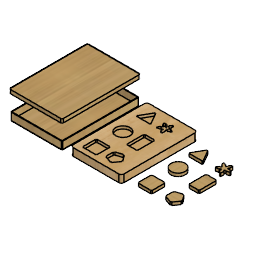
Modelação fushion_Parametrico (Autodesk Fusion 360 design; units mm, degrees)
Autodesk Fusion 360 part; units mm, degrees
sketch "Sketch1" plane through (0, 0, 0) normal (0, 1, 0) x (1, 0, 0)
sketch "Sketch2" plane through (0, 0, 0) normal (0, 0, 1) x (1, 0, 0)
  line L0 (0, 0) -> (-201, 0)
  line L1 (-201, 0) -> (-201, -301)
  line L2 (-201, -301) -> (0, -301)
  line L3 (0, -301) -> (0, 0)
  line L4 (1, -302) -> (1, 1)
  line L5 (1, 1) -> (-202, 1)
  line L6 (-202, 1) -> (-202, -302)
  line L7 (-202, -302) -> (1, -302)
  dimension "d11" = 201
  dimension "d12" = 301
  dimension "d13" = 1
  constraint horizontal L0
  constraint vertical L1
  constraint horizontal L2
  constraint vertical L3
  constraint coincident L0.start L3.end
  measures "d11" distance of L0.start L0.end
  measures "d12" distance of L0.start L2.end
extrude "Extrude1" add sketch "Sketch2" along normal blind 30 contours L0 L1 L2 L3 | L4 L5 L6 L7 makes body 1
fillet "Fillet1" radius 2.5 4 edges at (1, 1, 15) (1, -302, 15) (-202, 1, 15) (-202, -302, 15) on bodies 1
shell "Shell1" thickness 2.5 removed faces 1 at (-134.3333, -100.8333, 30) on bodies 1
sketch "Sketch3" plane through (0, 0, 30) normal (0, 0, 1) x (-1, 0, 0)
  line L0 (199.5, 1.5) -> (1.5, 1.5)
  line L1 (1.5, 1.5) -> (1.5, 299.5)
  line L2 (1.5, 299.5) -> (199.5, 299.5)
  line L3 (199.5, 299.5) -> (199.5, 1.5)
  arc A0 (202, 299.5) -> (199.5, 302) centre (199.5, 299.5) ccw
  line L4 (199.5, 302) -> (1.5, 302)
  arc A1 (1.5, 302) -> (-1, 299.5) centre (1.5, 299.5) ccw
  line L5 (-1, 299.5) -> (-1, 1.5)
  arc A2 (-1, 1.5) -> (1.5, -1) centre (1.5, 1.5) ccw
  line L6 (1.5, -1) -> (199.5, -1)
  arc A3 (199.5, -1) -> (202, 1.5) centre (199.5, 1.5) ccw
  line L7 (202, 1.5) -> (202, 299.5)
  line L8 (1.5, -4) -> (199.5, -4)
  arc A4 (199.5, -4) -> (205, 1.5) centre (199.5, 1.5) ccw
  line L9 (205, 1.5) -> (205, 299.5)
  arc A5 (205, 299.5) -> (199.5, 305) centre (199.5, 299.5) ccw
  line L10 (199.5, 305) -> (1.5, 305)
  arc A6 (1.5, 305) -> (-4, 299.5) centre (1.5, 299.5) ccw
  line L11 (-4, 299.5) -> (-4, 1.5)
  arc A7 (-4, 1.5) -> (1.5, -4) centre (1.5, 1.5) ccw
  dimension "d19" = 3
extrude "Extrude2" add sketch "Sketch3" against normal blind 15 from surface at 2.5 separate body contours L0 L1 L2 L3 | A0 L4 A1 L5 A2 L6 A3 L7 | L8 A4 L9 A5 L10 A6 L11 A7 makes body 2
shell "Shell2" thickness 2.5 removed faces 1 at (-65.6667, -100.8333, 17.5) on bodies 2
sketch "Sketch6" plane through (0, 0, 0) normal (0, 0, 1) x (1, 0, 0)
  line L0 (-0.4605, 150.568) -> (199.5395, 150.568)
  line L1 (199.5395, 150.568) -> (199.5395, -149.432)
  line L2 (199.5395, -149.432) -> (-0.4605, -149.432)
  line L3 (-0.4605, -149.432) -> (-0.4605, 150.568)
  dimension "d34" = 200
  dimension "d35" = 300
  constraint horizontal L0
  constraint vertical L1
  constraint horizontal L2
  constraint vertical L3
  measures "d34" distance of L0.start L0.end
  measures "d35" distance of L0.start L2.end
extrude "Extrude3" add sketch "Sketch6" along normal blind 30 separate body makes body 3
move_body "Move1" bodies 3 to x (1, 0, 0) y (0, 1, 0) z (0, 0, 1) at (33.944, 0, 0)
sketch "Sketch7" plane through (0, 0, 0) normal (0, 0, 1) x (1, 0, 0)
  line L0 (8, 0) -> (292, 0)
  line L1 (297, 8) -> (297, 202)
  line L2 (289, 210) -> (8, 210)
  line L3 (0, 202) -> (0, 8)
  arc A0 (0, 8) -> (8, 0) centre (8, 8) ccw
  arc A1 (289, 0) -> (297, 8) centre (289, 8) ccw
  arc A2 (297, 202) -> (289, 210) centre (289, 202) ccw
  arc A3 (8, 210) -> (0, 202) centre (8, 202) ccw
  dimension "d66" = 284
  dimension "d67" = 194
  measures "d66" horizontal distance of L0.start L0.end
  measures "d67" vertical distance of L1.start L1.end
extrude "Extrude4" add sketch "Sketch7" along normal blind 18 separate body makes body 4
ref_plane "WorkPlane1" through (0, 0, 18) normal (0, 0, 1) x (1, 0, 0)
sketch "Sketch8" plane through (0, 0, 18) normal (0, 0, 1) x (1, 0, 0)
  line L0 (18.5, 93.3) -> (74.3, 93.3)
  line L1 (74.3, 93.3) -> (74.3, 149.1)
  line L2 (74.3, 149.1) -> (18.5, 149.1)
  line L3 (18.5, 149.1) -> (18.5, 93.3)
  circle A0 centre (18.5, 93.3) radius 3.2
  circle A1 centre (74.3, 93.3) radius 3.2
  circle A2 centre (74.3, 149.1) radius 3.2
  circle A3 centre (18.5, 149.1) radius 3.2
  dimension "d71" = 55.8
  dimension "d72" = 55.8
  measures "d71" horizontal distance of L0.start L0.end
  measures "d72" vertical distance of L0.end L1.end
extrude "Extrude5" cut sketch "Sketch8" against normal blind 12.5 contours L0 L1 L2 L3 A0 A1 A2 A3 bodies 4
sketch "Sketch9" plane through (0, 0, 18) normal (0, 0, 1) x (1, 0, 0)
  circle A0 centre (118.2, 121.2) radius 28.4
  dimension "d75" = 28.4
  measures "d75" radius of A0
extrude "Extrude6" cut sketch "Sketch9" against normal blind 12.5 bodies 4
sketch "Sketch10" plane through (0, 0, 18) normal (0, 0, 1) x (1, 0, 0)
  line L0 (197, 155.1482) -> (167.6, 104.2259)
  line L1 (167.6, 104.2259) -> (226.4, 104.2259)
  line L2 (226.4, 104.2259) -> (197, 155.1482)
  circle A0 centre (197, 155.1482) radius 3.2
  circle A1 centre (167.6, 104.2259) radius 3.2
  circle A2 centre (226.4, 104.2259) radius 3.2
  dimension "d78" = 58.8
  dimension "d79" = 58.8
  dimension "d80" = 58.8
  measures "d78" distance of L0.start L0.end
  measures "d79" distance of L0.end L1.end
  measures "d80" distance of L1.end L0.start
extrude "Extrude7" cut sketch "Sketch10" against normal blind 12.5 contours L0 L1 L2 A0 A1 A2 bodies 4
sketch "Sketch11" plane through (0, 0, 18) normal (0, 0, 1) x (1, 0, 0)
  line L0 (276.8, 151.6) -> (269.3939, 131.3936)
  line L1 (269.3939, 131.3936) -> (247.8879, 130.5941)
  line L2 (247.8879, 130.5941) -> (264.8167, 117.3064)
  line L3 (264.8167, 117.3064) -> (258.9313, 96.6059)
  line L4 (258.9313, 96.6059) -> (276.8, 108.6)
  line L5 (276.8, 108.6) -> (294.6687, 96.6059)
  line L6 (294.6687, 96.6059) -> (288.7833, 117.3064)
  line L7 (288.7833, 117.3064) -> (305.7121, 130.5941)
  line L8 (305.7121, 130.5941) -> (284.2061, 131.3936)
  line L9 (284.2061, 131.3936) -> (276.8, 151.6)
  circle A0 centre (269.3939, 131.3936) radius 3.2
  circle A1 centre (264.8167, 117.3064) radius 3.2
  circle A2 centre (276.8, 108.6) radius 3.2
  circle A3 centre (288.7833, 117.3064) radius 3.2
  circle A4 centre (284.2061, 131.3936) radius 3.2
  line L10 (276.8, 121.2) -> (276.8, 151.6) construction
  line L11 (276.8, 121.2) -> (269.3939, 131.3936) construction
  dimension "d83" = 30.4
  dimension "d84" = 12.6
  measures "d83" distance of L10.start L0.start
  measures "d84" distance of L10.start L0.end
extrude "Extrude8" cut sketch "Sketch11" against normal blind 12.5 contours L0 L1 L2 L3 L4 L5 L6 L7 L8 L9 A0 A1 A2 A3 A4 bodies 4
sketch "Sketch12" plane through (0, 0, 18) normal (0, 0, 1) x (1, 0, 0)
  line L0 (46.4, 73.8) -> (19.39, 54.1761)
  line L1 (19.39, 54.1761) -> (29.7069, 22.4239)
  line L2 (29.7069, 22.4239) -> (63.0931, 22.4239)
  line L3 (63.0931, 22.4239) -> (73.41, 54.1761)
  line L4 (73.41, 54.1761) -> (46.4, 73.8)
  circle A0 centre (46.4, 73.8) radius 3.2
  circle A1 centre (19.39, 54.1761) radius 3.2
  circle A2 centre (29.7069, 22.4239) radius 3.2
  circle A3 centre (63.0931, 22.4239) radius 3.2
  circle A4 centre (73.41, 54.1761) radius 3.2
  line L5 (46.4, 45.4) -> (46.4, 73.8) construction
  dimension "d87" = 28.4
  measures "d87" distance of L5.start L0.start
extrude "Extrude9" cut sketch "Sketch12" against normal blind 12.5 contours L0 L1 L2 L3 L4 A0 A1 A2 A3 A4 bodies 4
sketch "Sketch13" plane through (0, 0, 18) normal (0, 0, 1) x (1, 0, 0)
  line L0 (118.2, 79.3482) -> (88.8, 28.4259)
  line L1 (88.8, 28.4259) -> (147.6, 28.4259)
  line L2 (147.6, 28.4259) -> (118.2, 79.3482)
  circle A0 centre (118.2, 79.3482) radius 3.2
  circle A1 centre (88.8, 28.4259) radius 3.2
  circle A2 centre (147.6, 28.4259) radius 3.2
  dimension "d90" = 58.8
  dimension "d91" = 58.8
  dimension "d92" = 58.8
  measures "d90" distance of L0.start L0.end
  measures "d91" distance of L0.end L1.end
  measures "d92" distance of L1.end L0.start
extrude "Extrude10" cut sketch "Sketch13" against normal blind 12.5 contours L0 L1 L2 A0 A1 A2 bodies 4
sketch "Sketch14" plane through (0, 0, 18) normal (0, 0, 1) x (1, 0, 0)
  line L0 (161.6, 24) -> (232.4, 24)
  line L1 (232.4, 24) -> (232.4, 66.8)
  line L2 (232.4, 66.8) -> (161.6, 66.8)
  line L3 (161.6, 66.8) -> (161.6, 24)
  circle A0 centre (161.6, 24) radius 3.2
  circle A1 centre (232.4, 24) radius 3.2
  circle A2 centre (232.4, 66.8) radius 3.2
  circle A3 centre (161.6, 66.8) radius 3.2
  dimension "d95" = 70.8
  dimension "d96" = 42.8
  measures "d95" horizontal distance of L0.start L0.end
  measures "d96" vertical distance of L0.end L1.end
extrude "Extrude11" cut sketch "Sketch14" against normal blind 12.5 contours L0 L1 L2 L3 A0 A1 A2 A3 bodies 4
sketch "Sketch15" plane through (0, 0, 18) normal (0, 0, 1) x (1, 0, 0)
  circle A0 centre (276.8, 45.4) radius 23.4
  dimension "d99" = 23.4
  measures "d99" radius of A0
extrude "Extrude12" cut sketch "Sketch15" against normal blind 12.5 bodies 4
sketch "Sketch16" plane through (0, 0, 18) normal (0, 0, 1) x (1, 0, 0)
  line L0 (2, 2) -> (10, 2)
  line L1 (10, 2) -> (10, 10)
  line L2 (10, 10) -> (2, 10)
  line L3 (2, 10) -> (2, 2)
  dimension "d102" = 8
  dimension "d103" = 8
  measures "d102" horizontal distance of L0.start L0.end
  measures "d103" vertical distance of L0.end L1.end
extrude "Extrude13" add sketch "Sketch16" along normal blind 6 bodies 4
sketch "Sketch17" plane through (0, 0, 18) normal (0, 0, 1) x (1, 0, 0)
  line L0 (287, 2) -> (295, 2)
  line L1 (295, 2) -> (295, 10)
  line L2 (295, 10) -> (287, 10)
  line L3 (287, 10) -> (287, 2)
  dimension "d106" = 8
  dimension "d107" = 8
  measures "d106" horizontal distance of L0.start L0.end
  measures "d107" vertical distance of L0.end L1.end
extrude "Extrude14" add sketch "Sketch17" along normal blind 6 bodies 4
sketch "Sketch18" plane through (0, 0, 18) normal (0, 0, 1) x (1, 0, 0)
  line L0 (2, 200) -> (10, 200)
  line L1 (10, 200) -> (10, 208)
  line L2 (10, 208) -> (2, 208)
  line L3 (2, 208) -> (2, 200)
  dimension "d110" = 8
  dimension "d111" = 8
  measures "d110" horizontal distance of L0.start L0.end
  measures "d111" vertical distance of L0.end L1.end
extrude "Extrude15" add sketch "Sketch18" along normal blind 6 bodies 4
sketch "Sketch19" plane through (0, 0, 18) normal (0, 0, 1) x (1, 0, 0)
  line L0 (287, 200) -> (295, 200)
  line L1 (295, 200) -> (295, 208)
  line L2 (295, 208) -> (287, 208)
  line L3 (287, 208) -> (287, 200)
  dimension "d114" = 8
  dimension "d115" = 8
  measures "d114" horizontal distance of L0.start L0.end
  measures "d115" vertical distance of L0.end L1.end
extrude "Extrude16" add sketch "Sketch19" along normal blind 6 bodies 4
ref_plane "WorkPlane2" through (0, 0, -6) normal (0, 0, 1) x (1, 0, 0)
sketch "Sketch20" plane through (0, 0, -6) normal (0, 0, 1) x (1, 0, 0)
  line L0 (15, 15) -> (35, 15)
  line L1 (35, 15) -> (35, 27)
  line L2 (35, 27) -> (15, 27)
  line L3 (15, 27) -> (15, 15)
  dimension "d119" = 20
  dimension "d120" = 12
  measures "d119" horizontal distance of L0.start L0.end
  measures "d120" vertical distance of L0.end L1.end
extrude "Extrude17" add sketch "Sketch20" along normal blind 6 bodies 4
sketch "Sketch21" plane through (0, 0, -6) normal (0, 0, 1) x (1, 0, 0)
  line L0 (262, 15) -> (282, 15)
  line L1 (282, 15) -> (282, 27)
  line L2 (282, 27) -> (262, 27)
  line L3 (262, 27) -> (262, 15)
  dimension "d123" = 20
  dimension "d124" = 12
  measures "d123" horizontal distance of L0.start L0.end
  measures "d124" vertical distance of L0.end L1.end
extrude "Extrude18" add sketch "Sketch21" along normal blind 6 bodies 4
sketch "Sketch22" plane through (0, 0, -6) normal (0, 0, 1) x (1, 0, 0)
  line L0 (15, 183) -> (35, 183)
  line L1 (35, 183) -> (35, 195)
  line L2 (35, 195) -> (15, 195)
  line L3 (15, 195) -> (15, 183)
  dimension "d127" = 20
  dimension "d128" = 12
  measures "d127" horizontal distance of L0.start L0.end
  measures "d128" vertical distance of L0.end L1.end
extrude "Extrude19" add sketch "Sketch22" along normal blind 6 bodies 4
sketch "Sketch23" plane through (0, 0, -6) normal (0, 0, 1) x (1, 0, 0)
  line L0 (262, 183) -> (282, 183)
  line L1 (282, 183) -> (282, 195)
  line L2 (282, 195) -> (262, 195)
  line L3 (262, 195) -> (262, 183)
  dimension "d131" = 20
  dimension "d132" = 12
  measures "d131" horizontal distance of L0.start L0.end
  measures "d132" vertical distance of L0.end L1.end
extrude "Extrude20" add sketch "Sketch23" along normal blind 6 bodies 4
ref_plane "WorkPlane3" through (0, 0, 2.3) normal (0, 0, 1) x (1, 0, 0)
sketch "Sketch24" plane through (0, 0, 2.3) normal (0, 0, 1) x (1, 0, 0)
  line L0 (327, 123.7) -> (382, 123.7)
  line L1 (382, 123.7) -> (382, 178.7)
  line L2 (382, 178.7) -> (327, 178.7)
  line L3 (327, 178.7) -> (327, 123.7)
  circle A0 centre (327, 123.7) radius 3.2
  circle A1 centre (382, 123.7) radius 3.2
  circle A2 centre (382, 178.7) radius 3.2
  circle A3 centre (327, 178.7) radius 3.2
  dimension "d136" = 55
  dimension "d137" = 55
  measures "d136" horizontal distance of L0.start L0.end
  measures "d137" vertical distance of L0.end L1.end
extrude "Extrude21" add sketch "Sketch24" along normal blind 12 separate body contours L0 L1 L2 L3 A0 A1 A2 A3 makes body 5
sketch "Sketch25" plane through (0, 0, 2.3) normal (0, 0, 1) x (1, 0, 0)
  circle A0 centre (424, 151.2) radius 28
  dimension "d140" = 28
  measures "d140" radius of A0
extrude "Extrude22" add sketch "Sketch25" along normal blind 12 separate body makes body 6
sketch "Sketch26" plane through (0, 0, 2.3) normal (0, 0, 1) x (1, 0, 0)
  line L0 (495, 184.6863) -> (466, 134.4568)
  line L1 (466, 134.4568) -> (524, 134.4568)
  line L2 (524, 134.4568) -> (495, 184.6863)
  circle A0 centre (495, 184.6863) radius 3.2
  circle A1 centre (466, 134.4568) radius 3.2
  circle A2 centre (524, 134.4568) radius 3.2
  dimension "d143" = 58
  dimension "d144" = 58
  dimension "d145" = 58
  measures "d143" distance of L0.start L0.end
  measures "d144" distance of L0.end L1.end
  measures "d145" distance of L1.end L0.start
extrude "Extrude23" add sketch "Sketch26" along normal blind 12 separate body contours L0 L1 L2 A0 A1 A2 makes body 7
sketch "Sketch27" plane through (0, 0, 2.3) normal (0, 0, 1) x (1, 0, 0)
  line L0 (568, 181.2) -> (560.3588, 161.7172)
  line L1 (560.3588, 161.7172) -> (539.4683, 160.4705)
  line L2 (539.4683, 160.4705) -> (555.6363, 147.1828)
  line L3 (555.6363, 147.1828) -> (550.3664, 126.9295)
  line L4 (550.3664, 126.9295) -> (568, 138.2)
  line L5 (568, 138.2) -> (585.6336, 126.9295)
  line L6 (585.6336, 126.9295) -> (580.3637, 147.1828)
  line L7 (580.3637, 147.1828) -> (596.5317, 160.4705)
  line L8 (596.5317, 160.4705) -> (575.6412, 161.7172)
  line L9 (575.6412, 161.7172) -> (568, 181.2)
  circle A0 centre (560.3588, 161.7172) radius 3.2
  circle A1 centre (555.6363, 147.1828) radius 3.2
  circle A2 centre (568, 138.2) radius 3.2
  circle A3 centre (580.3637, 147.1828) radius 3.2
  circle A4 centre (575.6412, 161.7172) radius 3.2
  line L10 (568, 151.2) -> (568, 181.2) construction
  line L11 (568, 151.2) -> (560.3588, 161.7172) construction
  dimension "d148" = 30
  dimension "d149" = 13
  measures "d148" distance of L10.start L0.start
  measures "d149" distance of L10.start L0.end
extrude "Extrude24" add sketch "Sketch27" along normal blind 12 separate body contours L0 L1 L2 L3 L4 L5 L6 L7 L8 L9 A0 A1 A2 A3 A4 makes body 8
sketch "Sketch28" plane through (0, 0, 2.3) normal (0, 0, 1) x (1, 0, 0)
  line L0 (355, 86.8) -> (328.3704, 67.4525)
  line L1 (328.3704, 67.4525) -> (338.542, 36.1475)
  line L2 (338.542, 36.1475) -> (371.458, 36.1475)
  line L3 (371.458, 36.1475) -> (381.6296, 67.4525)
  line L4 (381.6296, 67.4525) -> (355, 86.8)
  circle A0 centre (355, 86.8) radius 3.2
  circle A1 centre (328.3704, 67.4525) radius 3.2
  circle A2 centre (338.542, 36.1475) radius 3.2
  circle A3 centre (371.458, 36.1475) radius 3.2
  circle A4 centre (381.6296, 67.4525) radius 3.2
  line L5 (355, 58.8) -> (355, 86.8) construction
  dimension "d152" = 28
  measures "d152" distance of L5.start L0.start
extrude "Extrude25" add sketch "Sketch28" along normal blind 12 separate body contours L0 L1 L2 L3 L4 A0 A1 A2 A3 A4 makes body 9
sketch "Sketch29" plane through (0, 0, 2.3) normal (0, 0, 1) x (1, 0, 0)
  line L0 (426, 92.2863) -> (397, 42.0568)
  line L1 (397, 42.0568) -> (455, 42.0568)
  line L2 (455, 42.0568) -> (426, 92.2863)
  circle A0 centre (426, 92.2863) radius 3.2
  circle A1 centre (397, 42.0568) radius 3.2
  circle A2 centre (455, 42.0568) radius 3.2
  dimension "d155" = 58
  dimension "d156" = 58
  dimension "d157" = 58
  measures "d155" distance of L0.start L0.end
  measures "d156" distance of L0.end L1.end
  measures "d157" distance of L1.end L0.start
extrude "Extrude26" add sketch "Sketch29" along normal blind 12 separate body contours L0 L1 L2 A0 A1 A2 makes body 10
sketch "Sketch30" plane through (0, 0, 2.3) normal (0, 0, 1) x (1, 0, 0)
  line L0 (469, 37.8) -> (539, 37.8)
  line L1 (539, 37.8) -> (539, 79.8)
  line L2 (539, 79.8) -> (469, 79.8)
  line L3 (469, 79.8) -> (469, 37.8)
  circle A0 centre (469, 37.8) radius 3.2
  circle A1 centre (539, 37.8) radius 3.2
  circle A2 centre (539, 79.8) radius 3.2
  circle A3 centre (469, 79.8) radius 3.2
  dimension "d160" = 70
  dimension "d161" = 42
  measures "d160" horizontal distance of L0.start L0.end
  measures "d161" vertical distance of L0.end L1.end
extrude "Extrude27" add sketch "Sketch30" along normal blind 12 separate body contours L0 L1 L2 L3 A0 A1 A2 A3 makes body 11
sketch "Sketch31" plane through (0, 0, 2.3) normal (0, 0, 1) x (1, 0, 0)
  circle A0 centre (576, 58.8) radius 23
  dimension "d164" = 23
  measures "d164" radius of A0
extrude "Extrude28" add sketch "Sketch31" along normal blind 12 separate body makes body 12
move_body "Move2" bodies 4 to x (1, 0, 0) y (0, 1, 0) z (0, 0, 1) at (0, 189.5762, 0)
copy_body "CopyPasteBodies1" bodies 5 makes body 13
move_body "Move3" bodies 13 to x (1, 0, 0) y (0, 1, 0) z (0, 0, 1) at (-267.3879, -252.6694, 16)
copy_body "CopyPasteBodies2" bodies 6 makes body 14
move_body "Move4" bodies 14 to x (1, 0, 0) y (0, 1, 0) z (0, 0, 1) at (-336.8663, -179.3093, 25)
copy_body "CopyPasteBodies3" bodies 7 makes body 15
move_body "Move5" bodies 15 to x (1, 0, 0) y (0, 1, 0) z (0, 0, 1) at (-407.0549, -118.6328, 20)
move_body "Move6" bodies 15 to x (1, 0, 0) y (0, 1, 0) z (0, 0, 1) at (0, 54.0751, 0)
move_body "Move7" bodies 14 to x (1, 0, 0) y (0, 1, 0) z (0, 0, 1) at (0, 36.3001, 0)
move_body "Move8" bodies 15 to x (1, 0, 0) y (0, 1, 0) z (0, 0, 1) at (0, 12.4769, 0)
move_body "Move9" bodies 14 to x (1, 0, 0) y (0, 1, 0) z (0, 0, 1) at (0, -5.2559, 0)
copy_body "CopyPasteBodies4" bodies 9 makes body 16
move_body "Move10" bodies 16 to x (0, -1, 0) y (1, 0, 0) z (0, 0, 1) at (101.6321, 255.6253, 20)
copy_body "CopyPasteBodies5" bodies 11 makes body 17
move_body "Move11" bodies 17 to x (0, 1, 0) y (-1, 0, 0) z (0, 0, 1) at (217.6566, -502.3315, 20)
copy_body "CopyPasteBodies6" bodies 8 makes body 18
move_body "Move12" bodies 18 to x (0.965926, -0.258819, 0) y (0.258819, 0.965926, 0) z (0, 0, 1) at (-428.235, 99.4082, 20)
move_body "Move13" bodies 18 to x (0.998095, -0.06169, 0) y (0.06169, 0.998095, 0) z (0, 0, 1) at (-5.9386, 10.0808, 0)
move_body "Move14" bodies 14 to x (1, 0, 0) y (0, 1, 0) z (0, 0, 1) at (0, 0, -8)
move_body "Move15" bodies 13 to x (1, 0, 0) y (0, 1, 0) z (0, 0, 1) at (0, 0, 1)
move_body "Align1" bodies 15 to x (1, 0, 0) y (0, 1, 0) z (0, 0, 1) at (0, 0, -3)
move_body "Align2" bodies 18 to x (1, 0, 0) y (0, 1, 0) z (0, 0, 1) at (0, 0, -3)
move_body "Align3" bodies 17 to x (1, 0, 0) y (0, 1, 0) z (0, 0, 1) at (0, 0, -3)
move_body "Align4" bodies 16 to x (1, 0, 0) y (0, 1, 0) z (0, 0, 1) at (0, 0, -3)
move_body "Align5" bodies 13 to x (1, 0, 0) y (0, 1, 0) z (0, 0, 1) at (0, 0, 0)
combine "Combine1" operation cut target body 3 tool bodies 16 18 17
combine "Combine2" operation cut target body 3 tool bodies 14 13
combine "Combine3" operation cut target body 3 tool bodies 15
fillet "Fillet2" radius 10 4 edges at (233.4835, -149.432, 15) (233.4835, 150.568, 15) (33.4835, -149.432, 15) (33.4835, 150.568, 15) on bodies 3
move_body "Move16" bodies 2 to x (1, 0, 0) y (0, 1, 0) z (0, 0, 1) at (0, 0, 76.4154)
move_body "Move17" bodies 5 to x (1, 0, 0) y (0, 1, 0) z (0, 0, 1) at (-38.8932, -250.4721, 0)
move_body "Move18" bodies 6 to x (1, 0, 0) y (0, 1, 0) z (0, 0, 1) at (-108.6819, -145.659, 0)
move_body "Move19" bodies 7 to x (1, 0, 0) y (0, 1, 0) z (0, 0, 1) at (-180.2084, -59.6889, 0)
move_body "Move20" bodies 9 to x (0, -1, 0) y (1, 0, 0) z (0, 0, 1) at (351.8154, 253.813, 0)
move_body "Move21" bodies 11 to x (0, -1, 0) y (1, 0, 0) z (0, 0, 1) at (355.8753, 506.8384, 0)
move_body "Move22" bodies 8 to x (0.941239, -0.337742, 0) y (0.337742, 0.941239, 0) z (0, 0, 1) at (-176.3594, 143.3014, 0)
move_body "Move23" bodies 3 5 6 7 8 11 9 to x (1, 0, 0) y (0, 1, 0) z (0, 0, 1) at (0, -151.5069, 0)
move_body "Move24" bodies 5 6 7 9 11 8 to x (1, 0, 0) y (0, 1, 0) z (0, 0, 1) at (-13.312, 0, 0)
fillet "Fillet3" radius 2 5 edges at (426.0049, -58.6382, 8.3) (406.151, -29.4905, 8.3) (372.2946, -39.3655, 8.3) (371.2242, -74.6164, 8.3) (404.419, -86.5276, 8.3) on bodies 8
fillet "Fillet4" radius 3 5 edges at (134.9404, -70.4143, 24.65) (135.2708, -35.1487, 24.65) (168.9124, -24.5653, 24.65) (189.3737, -53.29, 24.65) (168.3778, -81.6262, 24.65) on bodies 3
hidden bodies 4 10 12
equation "Altura = 30 mm"
equation "compri = 200 mm"
equation "espassamento = 1 mm"
equation "tolerancia = 0.5 mm"
equation "Espessura = 2.5 mm"
equation "largura2 = 300 mm"
equation "alturadivisoria = 60 mm"
equation "d11 = compri + espassamento"
equation "d12 = largura2 + espassamento"
equation "d13 = espassamento"
equation "d14 = Altura"
equation "d17 = Espessura"
equation "d18 = Espessura"
equation "d19 = Espessura + tolerancia"
equation "d20 = Espessura"
equation "d23 = Espessura"
equation "circulo = 25 mm"
equation "quadrado = 30 mm"
equation "triangulo = 25 mm"
equation "semicirculo = 20 mm"
equation "trapezio = 30 mm"
equation "eclipse = 30 mm"
equation "d34 = compri"
equation "d35 = largura2"
equation "d36 = Altura"
equation "Largurabase = 300 mm"
equation "basealtura = 210.0 mm"
equation "Baseexpessurra = 18 mm"
equation "Raiocantobase = 8 mm"
equation "espessurapeças = 12 mm"
equation "profundidadecavidades = 12.5 mm"
equation "folgaporlado = 0.4 mm"
equation "quadradolado = 55 mm"
equation "circulogrande = 28 mm"
equation "triangulolado = 58 mm"
equation "Estrelaraioex = 30 mm"
equation "Estrelaraiointer = 13 mm"
equation "pentagonoraio = 28 mm"
equation "retangulolargura = 70 mm"
equation "retanguloaltura = 42 mm"
equation "circulopequeno = 23 mm"
equation "espaçoentrecolunas = 14 cm"
equation "espaçoentrelinhas = 16 mm"
equation "margemhorizontal = 18 mm"
equation "margemvertical = 16 mm"
equation "espaçoentrepeças = 14 mm"
equation "distanciabasepeças = 30 mm"
equation "ladopinoguia = 8 mm"
equation "alturapinoguia = 6 mm"
equation "comprimentope = 20 mm"
equation "largurape = 12 mm"
equation "alturape = 6 mm"
equation "d66 = Largurabase - 2 * Raiocantobase"
equation "d67 = basealtura - 2 * Raiocantobase"
equation "d68 = Baseexpessurra"
equation "d70 = Baseexpessurra"
equation "d71 = quadradolado + 2 * folgaporlado"
equation "d72 = quadradolado + 2 * folgaporlado"
equation "d73 = -( profundidadecavidades )"
equation "d75 = circulogrande + folgaporlado"
equation "d76 = -( profundidadecavidades )"
equation "d78 = triangulolado + 2 * folgaporlado"
equation "d79 = triangulolado + 2 * folgaporlado"
equation "d80 = triangulolado + 2 * folgaporlado"
equation "d81 = -( profundidadecavidades )"
equation "d83 = Estrelaraioex + folgaporlado"
equation "d84 = Estrelaraiointer - folgaporlado"
equation "d85 = -( profundidadecavidades )"
equation "d87 = pentagonoraio + folgaporlado"
equation "d88 = -( profundidadecavidades )"
equation "d90 = triangulolado + 2 * folgaporlado"
equation "d91 = triangulolado + 2 * folgaporlado"
equation "d92 = triangulolado + 2 * folgaporlado"
equation "d93 = -( profundidadecavidades )"
equation "d95 = retangulolargura + 2 * folgaporlado"
equation "d96 = retanguloaltura + 2 * folgaporlado"
equation "d97 = -( profundidadecavidades )"
equation "d99 = circulopequeno + folgaporlado"
equation "d100 = -( profundidadecavidades )"
equation "d102 = ladopinoguia"
equation "d103 = ladopinoguia"
equation "d104 = alturapinoguia"
equation "d106 = ladopinoguia"
equation "d107 = ladopinoguia"
equation "d108 = alturapinoguia"
equation "d110 = ladopinoguia"
equation "d111 = ladopinoguia"
equation "d112 = alturapinoguia"
equation "d114 = ladopinoguia"
equation "d115 = ladopinoguia"
equation "d116 = alturapinoguia"
equation "d118 = -alturape"
equation "d119 = comprimentope"
equation "d120 = largurape"
equation "d121 = alturape"
equation "d123 = comprimentope"
equation "d124 = largurape"
equation "d125 = alturape"
equation "d127 = comprimentope"
equation "d128 = largurape"
equation "d129 = alturape"
equation "d131 = comprimentope"
equation "d132 = largurape"
equation "d133 = alturape"
equation "d136 = quadradolado"
equation "d137 = quadradolado"
equation "d138 = espessurapeças"
equation "d140 = circulogrande"
equation "d141 = espessurapeças"
equation "d143 = triangulolado"
equation "d144 = triangulolado"
equation "d145 = triangulolado"
equation "d146 = espessurapeças"
equation "d148 = Estrelaraioex"
equation "d149 = Estrelaraiointer"
equation "d150 = espessurapeças"
equation "d152 = pentagonoraio"
equation "d153 = espessurapeças"
equation "d155 = triangulolado"
equation "d156 = triangulolado"
equation "d157 = triangulolado"
equation "d158 = espessurapeças"
equation "d160 = retangulolargura"
equation "d161 = retanguloaltura"
equation "d162 = espessurapeças"
equation "d164 = circulopequeno"
equation "d165 = espessurapeças"
equation "arrendodamento_base = 10 mm"
equation "d169 = arrendodamento_base"
named bodies: "Base", "Peca_Quadrado", "Peca_CirculoGrd", "Peca_Triangulo", "Peca_Estrela", "Peca_Pentagono", "Peca_Triangulo2", "Peca_Rectangulo", "Peca_CirculoPeq", "Peca_Quadrado (1)", "Peca_CirculoGrd (1)", "Peca_Triangulo (1)", "Peca_Pentagono (1)", "Peca_Rectangulo (1)", "Peca_Estrela (1)"
